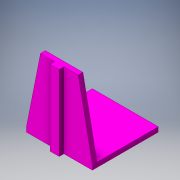
# Autodesk Inventor part: Bottom Elevator Bracket
Saved by Autodesk Inventor 2016 SP2 (Build 200236200, 236)
## iProperties
Created: 2018-01-27
Part Number: Bottom Elevator Bracket
Material: Generic
Document SubType Name: Modeling
Designer: CAD
Density: 1 g/cm^3
Appearance: Magenta
Author: CAD
Autodesk Inventor part; units mm, degrees
ref_plane "YZ Plane" through (0, 0, 0) normal (1, 0, 0) x (0, 1, 0)
ref_plane "XZ Plane" through (0, 0, 0) normal (0, 1, 0) x (-1, 0, 0)
ref_plane "XY Plane" through (0, 0, 0) normal (0, 0, 1) x (1, 0, 0)
sketch "Sketch1" plane through (0, 0, 0) normal (0, 1, 0) x (-1, 0, 0)
  line L0 (0, 0) -> (44.45, 0)
  line L1 (44.45, 0) -> (44.45, -44.45)
  line L2 (44.45, -44.45) -> (0, -44.45)
  line L3 (0, -44.45) -> (0, 0)
  dimension "d0" = 44.45
  dimension "d1" = 44.45
  constraints: 8 end point, 3 perpendicular, 1 horizontal
  measures "d0" distance of L0.start L0.end
  measures "d1" distance of L0.end L1.end
extrude "Extrusion1" add sketch "Sketch1" along normal blind 3.175
sketch "Sketch2" plane through (-44.45, 0, 0) normal (0, 0, 1) x (1, 0, 0)
  line L0 (9.525, 50.8) -> (34.925, 50.8)
  line L1 (44.45, 0) -> (0, 0) projected
  line L2 (22.225, 50.8) -> (22.225, 54.352)
  line L3 (22.225, 0) -> (22.225, -5.76)
  line L4 (9.525, 50.8) -> (0.0188, 3.175)
  line L5 (0.0188, 3.175) -> (44.4312, 3.175)
  line L6 (44.4312, 3.175) -> (34.925, 50.8)
  line L7 (0, 3.175) -> (44.45, 3.175) projected
  dimension "d4" = 25.4
  dimension "d5" = 50.8
  dimension "d6" = 0
  dimension "d9" = 0
  constraints: 12 end point, 2 horizontal, 2 midpoint, 2 vertical
  measures "d4" distance of L0.start L0.end
  measures "d5" distance between parallel lines of L1 L0
  measures "d6" distance between parallel lines of L2 L3
  measures "d9" distance between parallel lines of L7 L5
extrude "Extrusion2" add sketch "Sketch2" against normal blind 3.175
sketch "Sketch3" plane through (0, 0, 0) normal (0, -1, 0) x (1, 0, 0)
  line L0 (-25.273, 0) -> (-25.273, 3.175)
  line L1 (-19.177, 3.175) -> (-19.177, 0)
  line L2 (-19.177, 0) -> (-25.273, 0)
  line L3 (0, 0) -> (-44.45, 0) projected
  line L4 (-25.273, 3.175) -> (-19.177, 3.175)
  line L5 (0, -44.45) -> (0, 0) projected
  dimension "d10" = 3.175
  dimension "d13" = 6.096
  dimension "d14" = 19.177
  constraints: 8 end point, 1 collinear, 1 horizontal, 1 vertical
  measures "d10" distance of L0.start L0.end
  measures "d13" distance between parallel lines of L1 L0
  measures "d14" distance between parallel lines of L5 L1
extrude "Extrusion3" add sketch "Sketch3" against normal up to surface (50.8 mm away)
body "Solid1"
